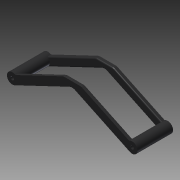
# Autodesk Inventor part: Front mount
Saved by Autodesk Inventor 2015 (Build 190159000, 159)
## iProperties
Created: 2016-10-31
Part Number: Front mount
Material: ABS Plastic
Document SubType Name: Modeling
Designer: James Yelland
Density: 1.06 g/cm^3
Appearance: Smooth - White
Mass: 7.98828 g
Surface Area: 62.2612 cm^2
Volume: 7.53611 cm^3
Author: James Yelland
Autodesk Inventor part; units mm, degrees
ref_plane "YZ Plane" through (0, 0, 0) normal (1, 0, 0) x (0, 1, 0)
ref_plane "XZ Plane" through (0, 0, 0) normal (0, 1, 0) x (-1, 0, 0)
ref_plane "XY Plane" through (0, 0, 0) normal (0, 0, 1) x (1, 0, 0)
sketch "Sketch2" plane through (0, 0, 0) normal (0, 1, 0) x (-1, 0, 0)
  circle A0 centre (50.479367, -84.432507) radius 1.4
  circle A1 centre (-50.479367, -84.432507) radius 1.4
  arc A2 (0, -65.970621) -> (-2.364635, -66.504889) centre (0, -71.470621) ccw
  arc A3 (2.364635, -66.504889) -> (0, -65.970621) centre (0, -71.470621) ccw
  line L0 (2.364635, -66.504889) -> (48.544666, -88.495379)
  line L1 (-2.364635, -66.504889) -> (-48.544666, -88.495379)
  arc A4 (48.544666, -88.495379) -> (47.928167, -80.725571) centre (50.479367, -84.432507) ccw
  arc A5 (-47.928167, -80.725571) -> (-48.544666, -88.495379) centre (-50.479367, -84.432507) ccw
  line L2 (-8.449668, -61.926286) -> (-47.928167, -80.725571)
  line L3 (8.449668, -61.926286) -> (47.928167, -80.725571)
  line L4 (-6.3, -61.440588) -> (6.3, -61.440588)
  arc A6 (-6.3, -61.440588) -> (-8.449668, -61.926286) centre (-6.3, -66.440588) ccw
  arc A7 (8.449668, -61.926286) -> (6.3, -61.440588) centre (6.3, -66.440588) ccw
  point P0 (0, 0)
  point P1 (52.5, -90.932667)
  dimension "d14" = 2.8
  dimension "d15" = 2.8
  dimension "d20" = 6.75
  dimension "d21" = 6.75
  dimension "d22" = 5
  constraints: 12 point on circle, 10 end point, 8 centre point, 4 tangent, 3 coincident, 1 equal radius, 1 horizontal
  measures "d14" diameter of A0
  measures "d15" diameter of A1
  measures "d20" distance between parallel lines of L1 L2
  measures "d21" distance between parallel lines of L3 L0
  measures "d22" radius of A6
extrude "Extrusion1" add sketch "Sketch2" along normal blind 3
sketch "Sketch3" plane through (0, 3, 0) normal (0, 1, 0) x (1, 0, 0)
  circle A0 centre (50.479367, 84.432507) radius 1.4
  circle A1 centre (-50.479367, 84.432507) radius 1.4
  line L0 (-2.364635, 66.504889) -> (-48.544666, 88.495379)
  arc A2 (-48.544666, 88.495379) -> (-47.928167, 80.725571) centre (-50.479367, 84.432507) ccw
  arc A3 (47.928167, 80.725571) -> (48.544666, 88.495379) centre (50.479367, 84.432507) ccw
  line L1 (48.544666, 88.495379) -> (2.364635, 66.504889)
  arc A4 (-2.364635, 66.504889) -> (2.364635, 66.504889) centre (0, 71.470621) ccw
  circle A5 centre (-50.479367, 84.432507) radius 1.4
  circle A6 centre (-50.479367, 84.432507) radius 4.5
  circle A7 centre (50.479367, 84.432507) radius 1.4
  circle A8 centre (50.479367, 84.432507) radius 4.5
  line L2 (-47.928167, 80.725571) -> (-8.449668, 61.926286)
  arc A9 (-8.449668, 61.926286) -> (-6.3, 61.440588) centre (-6.3, 66.440588) ccw
  line L3 (-6.3, 61.440588) -> (6.3, 61.440588)
  arc A10 (6.3, 61.440588) -> (8.449668, 61.926286) centre (6.3, 66.440588) ccw
  line L4 (8.449668, 61.926286) -> (47.928167, 80.725571)
  point P0 (0, 0)
  constraints: 4 centre point, 4 coincident, 4 concentric
extrude "Extrusion2" add sketch "Sketch3" along normal blind 24 contours A6 A2 | A3 A8
sketch "Sketch4" plane through (-50.479367, 27, -84.432507) normal (0, 1, 0) x (1, 0, 0)
  arc A0 (2.5512, -3.706936) -> (1.934701, 4.062872) centre (0, 0) ccw
  arc A1 (99.024032, 4.062872) -> (98.407533, -3.706936) centre (100.958733, 0) ccw
  line L0 (99.024032, 4.062872) -> (52.844001, -17.927619)
  arc A2 (48.114732, -17.927619) -> (52.844001, -17.927619) centre (50.479367, -12.961886) ccw
  line L1 (48.114732, -17.927619) -> (1.934701, 4.062872)
  circle A3 centre (0, 0) radius 4.5
  circle A4 centre (100.958733, 0) radius 1.4
  circle A5 centre (100.958733, 0) radius 4.5
  circle A6 centre (0, 0) radius 1.4
  line L2 (2.5512, -3.706936) -> (42.029699, -22.506222)
  arc A7 (42.029699, -22.506222) -> (44.179367, -22.991919) centre (44.179367, -17.991919) ccw
  line L3 (44.179367, -22.991919) -> (56.779367, -22.991919)
  arc A8 (56.779367, -22.991919) -> (58.929035, -22.506222) centre (56.779367, -17.991919) ccw
  line L4 (58.929035, -22.506222) -> (98.407533, -3.706936)
  point P0 (50.479367, -84.432507)
extrude "Extrusion3" add sketch "Sketch4" along normal blind 3
fillet "Fillet1" radius 1 17 edges at (-1.2121, 3, -66.1059) (1.2121, 3, -66.1059) (-25.4547, 3, -77.5001) (25.4547, 3, -77.5001) (0, 27, -65.9706) (25.4547, 27, -77.5001) (-25.4547, 27, -77.5001) (7.4019, 3, -61.5635) (28.1889, 3, -71.3259) (-7.4019, 3, -61.5635) (-28.1889, 3, -71.3259) (0, 3, -61.4406) (7.4019, 27, -61.5635) (28.1889, 27, -71.3259) (-7.4019, 27, -61.5635) (-28.1889, 27, -71.3259) (0, 27, -61.4406)
body "Solid1"
